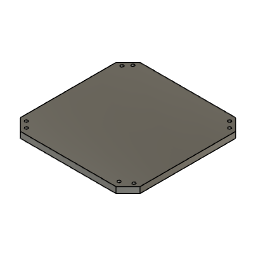
DroneBase v3 (Autodesk Fusion 360 design; units mm, degrees)
Autodesk Fusion 360 part; units mm, degrees
sketch "Sketch1" plane through (0, 0, 0) normal (0, 0, 1) x (1, 0, 0)
  line L0 (-80, 100) -> (80, 100)
  line L1 (100, 80) -> (100, -80)
  line L2 (80, -100) -> (-80, -100)
  line L3 (-100, -80) -> (-100, 80)
  line L4 (-80, 100) -> (-100, 80)
  line L5 (80, 100) -> (100, 80)
  line L6 (-80, -100) -> (-100, -80)
  line L7 (100, -80) -> (80, -100)
  circle A0 centre (90, 80) radius 2.5
  circle A1 centre (80, 90) radius 2.5
  circle A2 centre (-81.762, 90) radius 2.5
  circle A3 centre (-90, 80) radius 2.5
  circle A4 centre (-90, -80) radius 2.5
  circle A5 centre (-80, -90) radius 2.5
  circle A6 centre (75, -90) radius 2.5
  circle A7 centre (90, -80) radius 2.5
  point P0 (-100, 100)
  point P1 (100, 100)
  point P2 (100, -100)
  point P3 (-100, -100)
  dimension "d4" = 200
  dimension "d5" = 200
  dimension "d6" = 20
  dimension "d7" = 20
  dimension "d8" = 20
  dimension "d9" = 20
  dimension "d10" = 20
  dimension "d11" = 20
  dimension "d12" = 20
  dimension "d13" = 20
  dimension "d14" = 5
  dimension "d15" = 5
  dimension "d16" = 5
  dimension "d17" = 5
  dimension "d18" = 5
  dimension "d19" = 5
  dimension "d20" = 5
  dimension "d21" = 5
  constraint horizontal L0
  constraint vertical L1
  constraint horizontal L2
  constraint vertical L3
  constraint coincident P0 L0
  constraint coincident P0 L3
  constraint coincident P1 L0
  constraint coincident P1 L1
  constraint coincident P3 L2
  constraint coincident P3 L3
  constraint coincident P2 L1
  constraint coincident P2 L2
  measures "d4" distance of P0 P1
  measures "d5" distance of P0 P3
  measures "d6" distance of P0 L0.start
  measures "d7" distance of P0 L3.end
  measures "d8" distance of P1 L0.end
  measures "d9" distance of P1 L1.start
  measures "d10" distance of P3 L2.end
  measures "d11" distance of P3 L3.start
  measures "d12" distance of P2 L1.end
  measures "d13" distance of P2 L2.start
  measures "d14" diameter of A0
  measures "d15" diameter of A1
  measures "d16" diameter of A2
  measures "d17" diameter of A3
  measures "d18" diameter of A4
  measures "d19" diameter of A5
  measures "d20" diameter of A6
  measures "d21" diameter of A7
extrude "Extrude2" add sketch "Sketch1" along normal blind 10
extrude "Extrude1" [suppressed]
equation "d7 = d6"
equation "d9 = d8"
equation "d11 = d10"
equation "d13 = d12"
